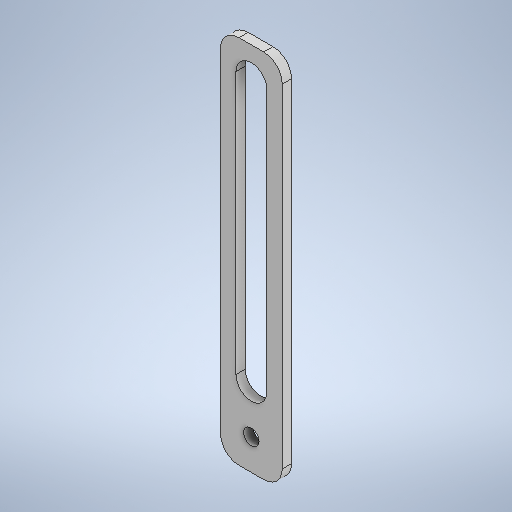
# Autodesk Inventor part: Eslabon 2
Saved by Autodesk Inventor 2025 (Build 290162000, 162)
## iProperties
Created: 2024-07-21
Part Number: Eslabon 2
Material: Genérico
Document SubType Name: Modeling
Designer: usuario
Density: 1 g/cm^3
Appearance: Valor por defecto
Author: usuario
Autodesk Inventor part; units mm, degrees
ref_plane "YZ Plane" through (0, 0, 0) normal (1, 0, 0) x (0, 1, 0)
ref_plane "XZ Plane" through (0, 0, 0) normal (0, 1, 0) x (-1, 0, 0)
ref_plane "XY Plane" through (0, 0, 0) normal (0, 0, 1) x (1, 0, 0)
sketch "Boceto1" plane through (0, 0, 0) normal (0, 0, 1) x (1, 0, 0)
  point P0 (0, 0)
sketch "Boceto2" plane through (0, 0, 0) normal (0, 0, 1) x (1, 0, 0)
  line L0 (12, 0) -> (28, 0)
  line L1 (40, 12) -> (40, 228)
  line L2 (28, 240) -> (12, 240)
  line L3 (0, 228) -> (0, 12)
  arc A0 (12, 240) -> (0, 228) centre (12, 228) ccw
  arc A1 (40, 228) -> (28, 240) centre (28, 228) ccw
  circle A2 centre (20, 20) radius 5
  line L4 (20, 40) -> (20, 40)
  line L5 (30, 50) -> (30, 220)
  line L6 (20, 230) -> (20, 230)
  line L7 (10, 220) -> (10, 50)
  line L8 (10, 40) -> (30, 230) construction
  line L9 (30, 40) -> (10, 230) construction
  arc A3 (0, 12) -> (12, 0) centre (12, 12) ccw
  arc A4 (28, 0) -> (40, 12) centre (28, 12) ccw
  arc A5 (10, 50) -> (20, 40) centre (20, 50) ccw
  arc A6 (20, 40) -> (30, 50) centre (20, 50) ccw
  arc A7 (20, 230) -> (10, 220) centre (20, 220) ccw
  arc A8 (30, 220) -> (20, 230) centre (20, 220) ccw
  point P0 (0, 0)
  point P1 (40, 240)
  point P2 (40, 0)
  point P3 (0, 240)
  point P4 (20, 0)
  point P5 (20, 135)
  point P6 (20, 40)
  point P7 (20, 230)
  point P8 (20, 240)
  dimension "d0" = 40
  dimension "d1" = 240
  dimension "d2" = 12
  dimension "d3" = 12
  dimension "d4" = 10
  dimension "d5" = 20
  dimension "d6" = 20
  dimension "d7" = 190
  dimension "d9" = 12
  dimension "d10" = 10
  dimension "d14" = 200
  constraints: 20 end point, 16 point on circle, 16 point on line, 16 tangent, 9 centre point, 4 equal radius, 4 midpoint, 4 parallel, 2 horizontal, 2 perpendicular
  measures "d0" distance of point (0, 240) point (40, 240)
  measures "d1" distance of point (40, 0) point (40, 240)
  measures "d2" radius of A0
  measures "d3" radius of A1
  measures "d4" diameter of A2
  measures "d5" distance of A2.centre point (20, 0)
  measures "d6" distance of L9.end L8.end
  measures "d7" distance of L8.end L9.start
  measures "d9" radius of A3
  measures "d10" radius of A5
  measures "d14" distance of A2.centre A7.centre
extrude "Extrusión1" add sketch "Boceto2" along normal blind 6
